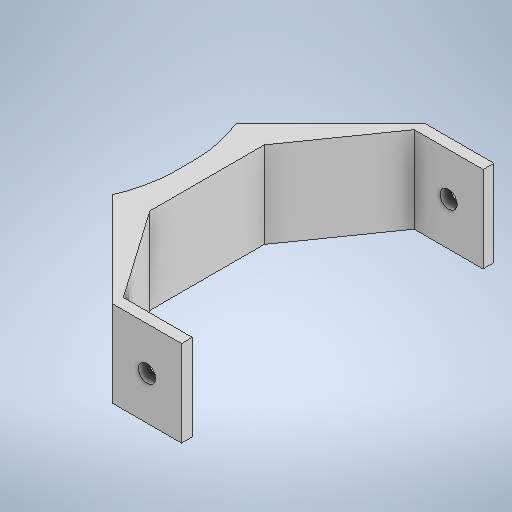
# Autodesk Inventor part: NeckRest
Saved by Autodesk Inventor 2025.1 (Build 291241000, 241)
## iProperties
Created: 2025-12-01
Part Number: NeckRest
Material: Generic
Document SubType Name: Modeling
Designer: Juxin
Density: 1 g/cm^3
Appearance: Default
Author: Juxin
Autodesk Inventor part; units mm, degrees
ref_plane "YZ Plane" through (0, 0, 0) normal (1, 0, 0) x (0, 1, 0)
ref_plane "XZ Plane" through (0, 0, 0) normal (0, 1, 0) x (-1, 0, 0)
ref_plane "XY Plane" through (0, 0, 0) normal (0, 0, 1) x (1, 0, 0)
sketch "Sketch1" plane through (0, 0, 0) normal (0, 1, 0) x (-1, 0, 0)
  line L0 (0, 0) -> (0, -46.0375)
  line L1 (0, 0) -> (20.32, 0)
  line L2 (20.32, 0) -> (20.32, -3.175)
  line L3 (20.32, -3.175) -> (0, -3.175)
  line L4 (0, -3.175) -> (0, 0)
  line L5 (0, -46.0375) -> (45.72, -46.0375)
  line L6 (0, -46.0375) -> (45.72, -46.0375) construction
  line L7 (45.72, -46.0375) -> (45.72, -39.6875)
  line L8 (64.77, -20.6375) -> (71.12, -20.6375)
  arc A0 (64.77, -20.6375) -> (45.72, -39.6875) centre (64.77, -39.6875) ccw
  line L9 (20.32, 0) -> (48.1588, -27.8388)
  line L10 (20.32, 0) -> (59.69, 0) construction
  line L11 (20.32, -3.175) -> (38.5311, -29.1831)
  line L12 (20.32, -3.175) -> (52.07, -3.175) construction
  line L13 (38.5311, -29.1831) -> (38.5311, -46.0375)
  arc A1 (48.1588, -27.8388) -> (44.9726, -46.0375) centre (86.9505, -44.0086) ccw
  line L14 (0, -92.075) -> (20.32, -92.075)
  line L15 (20.32, -88.9) -> (0, -88.9)
  line L16 (20.32, -92.075) -> (48.1588, -64.2362)
  line L17 (20.32, -88.9) -> (38.5311, -62.8919)
  line L18 (38.5311, -62.8919) -> (38.5311, -46.0375)
  arc A2 (44.9726, -46.0375) -> (48.1588, -64.2362) centre (86.9505, -48.0664) ccw
  line L19 (0, -92.075) -> (0, -88.9)
  point P0 (45.72, -20.6375)
  dimension "d1" = 20.32
  dimension "d5" = 45.72
  dimension "d6" = 0
  dimension "d8" = 25.4
  dimension "d9" = 25.4
  dimension "d12" = 19.05
  dimension "d13" = 39.37
  dimension "d14" = 45
  dimension "d15" = 31.75
  dimension "d16" = 55
  constraints: 40 end point, 7 symmetric about line, 6 horizontal, 6 point on circle, 4 point on line, 3 centre point, 3 equal length, 3 perpendicular, 2 parallel, 2 tangent, 2 vertical, 1 other
  measures "d1" distance of L2.end L3.end
  measures "d5" distance of L0.end L5.end
  measures "d6" distance between parallel lines of L5 L6
  measures "d8" distance of L6.end point (45.72, -20.637)
  measures "d9" distance of point (45.72, -20.637) L8.end
  measures "d12" radius of A0
  measures "d13" distance of L1.end L9.end
  measures "d14" angle of L9 L10
  measures "d15" distance of L2.end L11.end
  measures "d16" angle of L11 L12
extrude "Extrusion1" add sketch "Sketch1" along normal blind 25.4 contours L1 L2 L3 L0 | L9 A1 L5 L13 L11 L2 | L5 A2 L16 L14 L19 L15 L17 L18
sketch "Sketch2" plane through (-20.32, 0, 0) normal (0, 0, 1) x (1, 0, 0)
  line L0 (20.32, 0) -> (20.32, 25.4) projected
  line L1 (20.32, 12.7) -> (10.16, 12.7)
  circle A0 centre (10.16, 12.7) radius 2.54
  dimension "d19" = 10.16
  dimension "d20" = 5.08
  constraints: 2 end point, 1 centre point, 1 coincident, 1 horizontal, 1 midpoint
  measures "d19" distance of L1.start L1.end
  measures "d20" diameter of A0
extrude "Extrusion2" cut sketch "Sketch2" against normal blind 142.875
body "Solid1"
